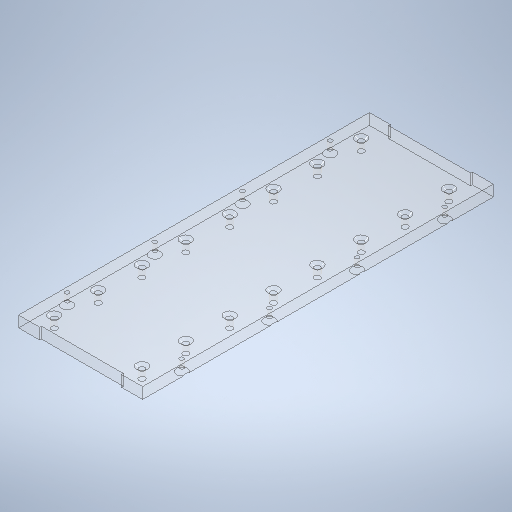
# Autodesk Inventor part: Base V1
Saved by Autodesk Inventor 2025 (Build 290162000, 162)
## iProperties
Created: 2024-03-20
Part Number: Base V1
Material: PMMA Plastic
Document SubType Name: Modeling
Designer: cfang
Density: 1.188 g/cm^3
Appearance: Polycarbonate - Clear
Author: cfang
Autodesk Inventor part; units mm, degrees
ref_plane "YZ Plane" through (0, 0, 0) normal (1, 0, 0) x (0, 1, 0)
ref_plane "XZ Plane" through (0, 0, 0) normal (0, 1, 0) x (-1, 0, 0)
ref_plane "XY Plane" through (0, 0, 0) normal (0, 0, 1) x (1, 0, 0)
sketch "Sketch1" plane through (0, 0, 0) normal (0, 1, 0) x (-1, 0, 0)
  line L0 (-35.35, -100) -> (35.35, -100)
  line L1 (35.35, -100) -> (35.35, 100)
  line L2 (35.35, 100) -> (-35.35, 100)
  line L3 (-35.35, 100) -> (-35.35, -100)
  line L4 (-35.35, -100) -> (35.35, 100) construction
  line L5 (35.35, -100) -> (-35.35, 100) construction
  point P0 (0, 0)
  dimension "d0" = 200
  dimension "d1" = 70.7
  constraints: 12 end point, 2 midpoint, 2 parallel, 1 horizontal, 1 perpendicular
  measures "d0" distance of L0.end L1.end
  measures "d1" distance of L1.end L2.end
extrude "Extrusion1" add sketch "Sketch1" along normal blind 6.35
sketch "Sketch2" plane through (0, 6.35, 0) normal (0, 1, 0) x (1, 0, 0)
  line L0 (-35.35, -100) -> (35.35, -100) projected
  line L1 (-35.35, 100) -> (-35.35, -100) projected
  point P0 (0, 0)
  point P1 (-25, -90)
  point P2 (25, -90)
  point P3 (-25, -65)
  point P4 (25, -65)
  point P5 (-25, -40)
  point P6 (25, -40)
  point P7 (-25, -15)
  point P8 (25, -15)
  point P9 (-25, 10)
  point P10 (25, 10)
  point P11 (-25, 35)
  point P12 (25, 35)
  point P13 (-25, 60)
  point P14 (25, 60)
  point P15 (-25, 85)
  point P16 (25, 85)
  dimension "d4" = 50
  dimension "d5" = 25
  dimension "d6" = 10
  dimension "d9" = 25
  constraints: 1 horizontal alignment, 1 vertical, 14 other
  measures "d4" distance of point (-25, -90) point (25, -90)
  measures "d5" horizontal distance of point (-25, -90) point (0, 0)
  measures "d6" distance from line of L0 point (-25, -90)
  measures "d9" distance of point (-25, -90) point (-25, -65)
hole "Hole1" at (-25, 6.35, 90) at (25, 6.35, 90) at (-25, 6.35, 65) at (25, 6.35, 65) at (-25, 6.35, 40) at (25, 6.35, 40) at (-25, 6.35, 15) at (25, 6.35, 15) at (-25, 6.35, -10) at (25, 6.35, -10) at (-25, 6.35, -35) at (25, 6.35, -35) at (-25, 6.35, -60) at (25, 6.35, -60) at (-25, 6.35, -85) at (25, 6.35, -85) direction (0, -1, 0) diameter 3.4 end through all countersink diameter 6.3 countersink angle 90 clearance for "Flat Head Machine Screw" size "M3" standard "Ansi Metric M Profile"
sketch "Sketch5" plane through (-35.35, 0, 100) normal (0, 0, 1) x (1, 0, 0)
  line L0 (0, 0) -> (70.7, 0) projected
  line L1 (70.7, 6.35) -> (0, 6.35) projected
  line L2 (12, 0) -> (58.7, 0)
  line L3 (58.7, 0) -> (58.7, 6.35)
  line L4 (58.7, 6.35) -> (12, 6.35)
  line L5 (12, 6.35) -> (12, 0)
  line L6 (0, 0) -> (0, 6.35) projected
  line L7 (70.7, 0) -> (70.7, 6.35) projected
  point P0 (35.35, 0)
  point P1 (12, 6.35)
  dimension "d37" = 12
  dimension "d38" = 12
  constraints: 8 end point, 2 parallel, 2 point on line, 1 horizontal, 1 perpendicular
  measures "d37" distance between parallel lines of L6 L5
  measures "d38" distance between parallel lines of L7 L3
extrude "Extrusion3" cut sketch "Sketch5" against normal blind 1 contours L5 L1 L3 L0
sketch "Sketch6" plane through (35.35, 0, -100) normal (0, 0, -1) x (-1, 0, 0)
  line L0 (58.7, 6.35) -> (12, 6.35) projected
  line L1 (12, -1.35) -> (58.7, -1.35)
  line L2 (58.7, -1.35) -> (58.7, 6.35)
  line L3 (58.7, 6.35) -> (12, 6.35)
  line L4 (12, 6.35) -> (12, -1.35)
  line L5 (0, 0) -> (0, 6.35) projected
  line L6 (70.7, 0) -> (70.7, 6.35) projected
  point P0 (35.35, 0)
  point P1 (12, 2.5)
  point P2 (12, 6.35)
  dimension "d41" = 12
  dimension "d42" = 12
  constraints: 8 end point, 2 parallel, 1 horizontal, 1 midpoint, 1 perpendicular, 1 point on line
  measures "d41" distance from line of L5 point (12, 2.5)
  measures "d42" distance between parallel lines of L6 L2
extrude "Extrusion4" cut sketch "Sketch6" against normal blind 1
sketch "Sketch7" plane through (0, 0, 0) normal (0, -1, 0) x (1, 0, 0)
  line L0 (35.35, 100) -> (35.35, -100) projected
  line L1 (-35.35, -100) -> (-35.35, 100) projected
  point P0 (0, 0)
  point P1 (32.675, 25)
  point P2 (32.675, 75)
  point P3 (32.675, -25)
  point P4 (32.675, -75)
  point P5 (-32.675, 75)
  point P6 (-32.675, 25)
  point P7 (-32.675, -25)
  point P8 (-32.675, -75)
  dimension "d45" = 25
  dimension "d46" = 2.675
  dimension "d47" = 25
  dimension "d48" = 50
  dimension "d49" = 50
  dimension "d50" = 2.675
  constraints: 6 vertical alignment, 4 horizontal alignment
  measures "d45" vertical distance of point (32.675, 25) point (0, 0)
  measures "d46" distance from line of L0 point (32.675, 25)
  measures "d47" vertical distance of point (32.675, -25) point (0, 0)
  measures "d48" distance of point (32.675, -75) point (32.675, -25)
  measures "d49" distance of point (32.675, 75) point (32.675, 25)
  measures "d50" distance from line of L1 point (-32.675, 75)
hole "Hole3" at (32.675, 0, 25) at (32.675, 0, 75) at (32.675, 0, -25) at (32.675, 0, -75) at (-32.675, 0, 75) at (-32.675, 0, 25) at (-32.675, 0, -25) at (-32.675, 0, -75) direction (0, 1, 0) diameter 2.4 depth 10 tip angle 118 countersink diameter 6.3 countersink angle 90 clearance for "Flat Head Machine Screw" size "M2" standard "Ansi Metric M Profile"
equation "\"d5\" = 0.5 * d4"
equation "\"d47\" = d45"
equation "\"d48\" = 2 * d47"
equation "\"d49\" = d48"
equation "\"d50\" = d46"
body "Solid1"
